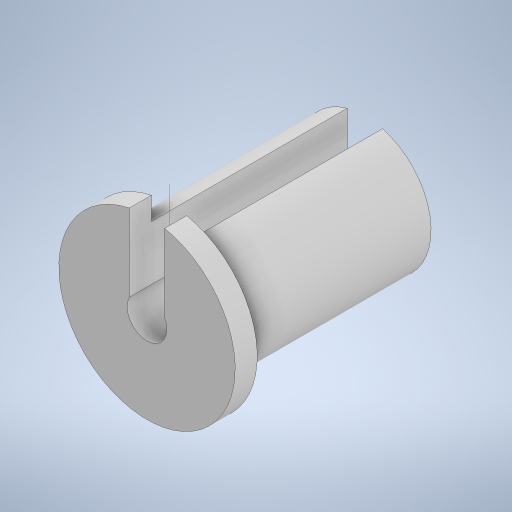
# Autodesk Inventor part: wallPlug
Saved by Autodesk Inventor 2023 (Build 270158030, 158C)
## iProperties
Created: 2022-06-04
Part Number: wallPlug
Material: Generic
Document SubType Name: Modeling
Designer: snobo
Density: 1 g/cm^3
Appearance: Default
Author: snobo
Autodesk Inventor part; units mm, degrees
ref_plane "YZ Plane" through (0, 0, 0) normal (1, 0, 0) x (0, 1, 0)
ref_plane "XZ Plane" through (0, 0, 0) normal (0, 1, 0) x (-1, 0, 0)
ref_plane "XY Plane" through (0, 0, 0) normal (0, 0, 1) x (1, 0, 0)
sketch "Sketch1" plane through (0, 0, 0) normal (0, 0, 1) x (1, 0, 0)
  circle A0 centre (0, 0) radius 20
  dimension "d0" = 40
  constraints: 1 centre point, 1 coincident
  measures "d0" diameter of A0
extrude "Extrusion1" add sketch "Sketch1" along normal blind 5
sketch "Sketch2" plane through (0, 0, 0) normal (0, 0, -1) x (-1, 0, 0)
  circle A0 centre (0, 0) radius 15
  dimension "d3" = 30
  constraints: 1 centre point, 1 coincident
  measures "d3" diameter of A0
extrude "Extrusion2" add sketch "Sketch2" along normal blind 44.45
sketch "Sketch3" plane through (0, 0, 5) normal (0, 0, 1) x (1, 0, 0)
  circle A0 centre (0, 0) radius 4.5
  dimension "d6" = 9
  constraints: 1 centre point, 1 coincident
  measures "d6" diameter of A0
extrude "Extrusion3" cut sketch "Sketch3" against normal through all
sketch "Sketch4" plane through (0, 0, 5) normal (0, 0, 1) x (1, 0, 0)
  circle A0 centre (0, 0) radius 4.5 projected
  line L0 (-4, 2.0616) -> (-4, 19.5959)
  circle A1 centre (0, 0) radius 20 projected
  line L1 (4, 2.0616) -> (4, 19.5959)
  line L2 (0, -28) -> (0, 28) projected
  arc A2 (4, 2.0616) -> (-4, 2.0616) centre (0, 0) ccw
  arc A3 (0, -20) -> (-4, 19.5959) centre (0, 0) ccw
  dimension "d11" = 4
  constraints: 8 point on circle, 4 end point, 2 centre point, 2 coincident, 2 concentric, 2 parallel, 1 point on line, 1 vertical
  measures "d11" distance between parallel lines of L2 L0
extrude "Extrusion4" cut sketch "Sketch4" against normal through all contours A0 L2 A1 L1 | A0 L0 A1 L2 picked at (1.3394, 14.7583) picked at (-1.3394, 14.7583)
body "Solid1"
